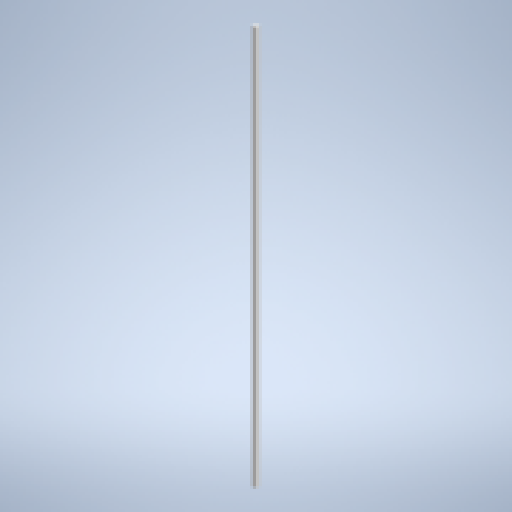
# Autodesk Inventor part: auxiliar
Saved by Autodesk Inventor 2024 (Build 280153000, 153)
## iProperties
Created: 2024-04-21
Part Number: auxiliar
Material: Genérico
Document SubType Name: Modeling
Designer: sergi
Density: 1 g/cm^3
Appearance: Valor por defecto
Author: sergi
Autodesk Inventor part; units mm, degrees
ref_plane "YZ Plane" through (0, 0, 0) normal (1, 0, 0) x (0, 1, 0)
ref_plane "XZ Plane" through (0, 0, 0) normal (0, 1, 0) x (-1, 0, 0)
ref_plane "XY Plane" through (0, 0, 0) normal (0, 0, 1) x (1, 0, 0)
sketch "Boceto1" plane through (0, 0, 0) normal (0, 1, 0) x (-1, 0, 0)
  line L0 (-0.05, 0.05) -> (0.05, 0.05)
  line L1 (0.05, 0.05) -> (0.05, -0.05)
  line L2 (0.05, -0.05) -> (-0.05, -0.05)
  line L3 (-0.05, -0.05) -> (-0.05, 0.05)
  line L4 (-0.05, 0.05) -> (0.05, -0.05) construction
  line L5 (0.05, 0.05) -> (-0.05, -0.05) construction
  point P0 (0, 0)
  dimension "d0" = 0.1
  dimension "d1" = 0.1
  constraints: 12 end point, 2 midpoint, 2 parallel, 1 horizontal, 1 perpendicular
  measures "d0" distance of L1.end L2.end
  measures "d1" distance of L0.end L1.end
extrude "Extrusión1" add sketch "Boceto1" along normal blind 100
